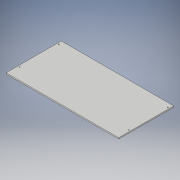
# Autodesk Inventor part: wall-front-outer
Saved by Autodesk Inventor 2017 (Build 210142000, 142)
## iProperties
Created: 2017-02-28
Part Number: wall-front-outer
Material: Generic
Document SubType Name: Modeling
Designer: John
Density: 1 g/cm^3
Appearance: Default
Author: John
Autodesk Inventor part; units mm, degrees
ref_plane "YZ Plane" through (0, 0, 0) normal (1, 0, 0) x (0, 1, 0)
ref_plane "XZ Plane" through (0, 0, 0) normal (0, 1, 0) x (-1, 0, 0)
ref_plane "XY Plane" through (0, 0, 0) normal (0, 0, 1) x (1, 0, 0)
sketch "Sketch1" plane through (0, 0, 0) normal (0, 1, 0) x (-1, 0, 0)
  line L0 (0, 0) -> (286, 0)
  line L1 (286, 0) -> (286, 140)
  line L2 (286, 140) -> (0, 140)
  line L3 (0, 140) -> (0, 0)
  circle A0 centre (4.25, 10.75) radius 1.25
  circle A1 centre (4.25, 110.25) radius 1.25
  line L4 (143, 140) -> (143, 0) construction
  circle A2 centre (281.75, 10.75) radius 1.25
  circle A3 centre (281.75, 110.25) radius 1.25
  dimension "d0" = 286
  dimension "d1" = 140
  dimension "d4" = 2.5
  dimension "d5" = 4.25
  dimension "d6" = 10.75
  dimension "d7" = 2.5
  dimension "d8" = 4.25
  dimension "d9" = 99.5
  constraints: 10 end point, 4 centre point, 2 midpoint, 2 parallel, 2 symmetric about line, 1 horizontal, 1 perpendicular, 2 other
  measures "d0" distance of L2.end L1.end
  measures "d1" distance of L1.end L0.end
  measures "d4" diameter of A0
  measures "d5" distance from line of L3 A0.centre
  measures "d6" distance from line of L0 A0.centre
  measures "d7" diameter of A1
  measures "d8" distance from line of L3 A1.centre
  measures "d9" distance of A0.centre A1.centre
extrude "Extrusion1" add sketch "Sketch1" along normal blind 3
equation "\"d7\" = d4"
equation "\"d8\" = d5"
body "Solid1"
